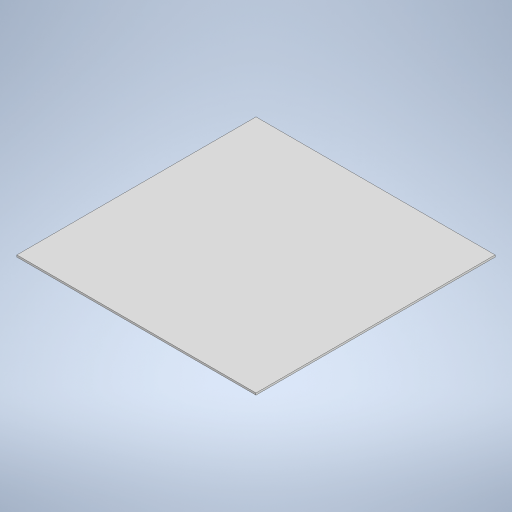
# Autodesk Inventor part: Cuadricula
Saved by Autodesk Inventor 2024.2 (Build 282272000, 272)
## iProperties
Created: 2024-07-18
Part Number: Cuadricula
Material: Generic
Document SubType Name: Modeling
Designer: jrcer
Density: 1 g/cm^3
Appearance: Default
Author: jrcer
Autodesk Inventor part; units mm, degrees
ref_plane "YZ Plane" through (0, 0, 0) normal (1, 0, 0) x (0, 1, 0)
ref_plane "XZ Plane" through (0, 0, 0) normal (0, 1, 0) x (-1, 0, 0)
ref_plane "XY Plane" through (0, 0, 0) normal (0, 0, 1) x (1, 0, 0)
sketch "Sketch1" plane through (0, 0, 0) normal (0, 1, 0) x (-1, 0, 0)
  line L0 (205, 205) -> (-205, 205)
  line L1 (-205, 205) -> (-205, -205)
  line L2 (-205, -205) -> (205, -205)
  line L3 (205, -205) -> (205, 205)
  line L4 (205, 205) -> (-205, -205) construction
  line L5 (-205, 205) -> (205, -205) construction
  point P0 (0, 0)
  dimension "d0" = 410
  dimension "d1" = 410
  constraints: 12 end point, 2 midpoint, 2 parallel, 1 horizontal, 1 perpendicular
  measures "d0" distance of L2.end L1.end
  measures "d1" distance of L1.end L0.end
extrude "Extrusion1" add sketch "Sketch1" along normal blind 3.25
body "Solid1"
